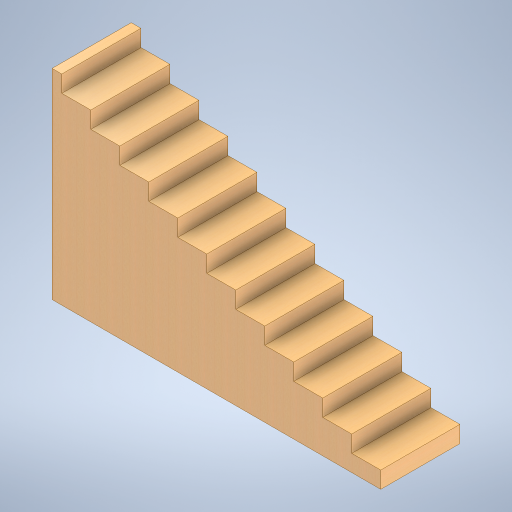
# Autodesk Inventor part: Stairs_Between_Basement_And_First_Floor
Saved by Autodesk Inventor 2024 (Build 280153000, 153)
## iProperties
Created: 2023-05-16
Part Number: Stairs_Between_Basement_And_First_Floor
Material: Wood (Oak)
Document SubType Name: Modeling
Designer: Tom
Density: 0.76 g/cm^3
Appearance: Yellow Pine - Solid Stained Light Low Gloss
Author: Tom
Autodesk Inventor part; units mm, degrees
ref_plane "YZ Plane" through (0, 0, 0) normal (1, 0, 0) x (0, 1, 0)
ref_plane "XZ Plane" through (0, 0, 0) normal (0, 1, 0) x (-1, 0, 0)
ref_plane "XY Plane" through (0, 0, 0) normal (0, 0, 1) x (1, 0, 0)
sketch "Sketch1" plane through (0, 0, 0) normal (0, 0, 1) x (1, 0, 0)
  line L0 (0, 0) -> (0, 184.6792)
  line L1 (0, 184.6792) -> (-320.9636, 184.6792)
  line L2 (-320.9636, 184.6792) -> (-320.9636, 369.3583)
  line L3 (-320.9636, 369.3583) -> (-641.9273, 369.3583)
  line L4 (-641.9273, 369.3583) -> (-641.9273, 554.0375)
  line L5 (-641.9273, 554.0375) -> (-962.8909, 554.0375)
  line L6 (-962.8909, 554.0375) -> (-962.8909, 738.7167)
  line L7 (-962.8909, 738.7167) -> (-1283.8545, 738.7167)
  line L8 (-1283.8545, 738.7167) -> (-1283.8545, 923.3958)
  line L9 (-1283.8545, 923.3958) -> (-1604.8182, 923.3958)
  line L10 (-1604.8182, 923.3958) -> (-1604.8182, 1108.075)
  line L11 (-1604.8182, 1108.075) -> (-1925.7818, 1108.075)
  line L12 (-1925.7818, 1108.075) -> (-1925.7818, 1292.7542)
  line L13 (-1925.7818, 1292.7542) -> (-2246.7455, 1292.7542)
  line L14 (-2246.7455, 1292.7542) -> (-2246.7455, 1477.4333)
  line L15 (-2246.7455, 1477.4333) -> (-2567.7091, 1477.4333)
  line L16 (-2567.7091, 1477.4333) -> (-2567.7091, 1662.1125)
  line L17 (-2567.7091, 1662.1125) -> (-2888.6727, 1662.1125)
  line L18 (-2888.6727, 1662.1125) -> (-2888.6727, 1846.7917)
  line L19 (-2888.6727, 1846.7917) -> (-3209.6364, 1846.7917)
  line L20 (-3209.6364, 1846.7917) -> (-3209.6364, 2031.4708)
  line L21 (-3209.6364, 2031.4708) -> (-3530.6, 2031.4708)
  line L22 (-3530.6, 2031.4708) -> (-3530.6, 2216.15)
  line L23 (-3530.6, 2216.15) -> (-3638.55, 2216.15)
  line L24 (-3638.55, 2216.15) -> (-3638.55, 0)
  line L25 (-3638.55, 0) -> (0, 0)
  dimension "d2" = 3530.6
  dimension "d3" = 107.95
  dimension "d6" = 2216.15
  constraints: 52 end point, 23 perpendicular, 21 parallel, 2 horizontal, 1 vertical
  measures "d2" horizontal distance of L0.start L22.end
  measures "d3" distance between parallel lines of L24 L22
  measures "d6" distance of L23.end L24.end
extrude "Extrusion1" add sketch "Sketch1" along normal blind 876.3
body "Solid1"
